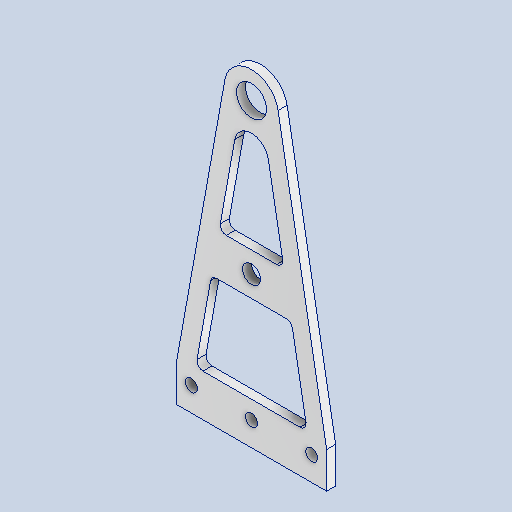
# Autodesk Inventor part: 1171
Saved by Autodesk Inventor 2025.1 (Build 291241000, 241)
## iProperties
Created: 2024-06-11
Part Number: 1171
Material: Aluminium 6061
Document SubType Name: Modeling
Designer: ffogue
Density: 2.7 g/cm^3
Appearance: Aluminium - flach
Author: ffogue
Autodesk Inventor part; units mm, degrees
ref_plane "YZ Plane" through (0, 0, 0) normal (1, 0, 0) x (0, 1, 0)
ref_plane "XZ Plane" through (0, 0, 0) normal (0, 1, 0) x (-1, 0, 0)
ref_plane "XY Plane" through (0, 0, 0) normal (0, 0, 1) x (1, 0, 0)
sketch "Skizze1" plane through (0, 0, 0) normal (0, 1, 0) x (-1, 0, 0)
  line L0 (25, 0) -> (-25, 0)
  line L1 (-25, 0) -> (-25, 12)
  line L2 (-25, 12) -> (-8.8574, 101.5958)
  arc A0 (8.8574, 101.5958) -> (-8.8574, 101.5958) centre (0, 100) ccw
  line L3 (8.8574, 101.5958) -> (25, 12)
  line L4 (25, 12) -> (25, 0)
  line L5 (0, 100) -> (0, 0) construction
  dimension "d0" = 100
  dimension "d1" = 12
  dimension "d2" = 50
  dimension "d3" = 9
  constraints: 12 end point, 2 point on circle, 1 centre point, 1 horizontal, 1 horizontal alignment, 1 midpoint, 1 parallel, 1 perpendicular, 1 symmetric about line, 1 tangent, 1 vertical, 1 vertical alignment
  measures "d0" distance of L5.start L5.end
  measures "d1" distance of L0.end L1.end
  measures "d2" distance of L0.start L0.end
  measures "d3" radius of A0
extrude "Extrusion1" add sketch "Skizze1" along normal blind 3
sketch "Skizze3" plane through (0, 3, 0) normal (0, 1, 0) x (1, 0, 0)
  arc A0 (-8.8574, -101.5958) -> (8.8574, -101.5958) centre (0, -100) ccw projected
  point P0 (0, 0)
  point P1 (0, -100)
  constraints: 1 coincident
hole "Bohrung1" at (0, 3, 100) direction (0, -1, 0) diameter 10 depth 3
sketch "Skizze4" plane through (0, 3, 0) normal (0, 1, 0) x (1, 0, 0)
  line L0 (-10.7957, -57) -> (10.7957, -57)
  line L1 (10.7957, -57) -> (5.5701, -86.0036)
  arc A0 (-5.5701, -86.0036) -> (5.5701, -86.0036) centre (0, -85) ccw
  line L2 (-5.5701, -86.0036) -> (-10.7957, -57)
  line L3 (25, 0) -> (-25, 0) projected
  line L4 (8.8574, -101.5958) -> (25, -12) projected
  line L5 (-25, -12) -> (-8.8574, -101.5958) projected
  circle A1 centre (0, -100) radius 5 projected
  point P0 (0, 0)
  point P1 (0, 0)
  dimension "d13" = 15
  dimension "d14" = 6
  dimension "d15" = 43
  constraints: 6 end point, 2 parallel, 2 point on circle, 1 centre point, 1 horizontal, 1 horizontal alignment, 1 midpoint, 1 tangent, 1 vertical alignment
  measures "d13" distance of A1.centre A0.centre
  measures "d14" distance between parallel lines of L5 L2
  measures "d15" distance from line of L0 A1.centre
extrude "Extrusion2" cut sketch "Skizze4" against normal up to surface (3 mm away) contours L0 L1 A0 L2
sketch "Skizze5" plane through (0, 3, 0) normal (0, 1, 0) x (1, 0, 0)
  line L0 (13.3181, -43) -> (-13.3181, -43)
  line L1 (-13.3181, -43) -> (-18.543, -14)
  line L2 (-18.543, -14) -> (18.543, -14)
  line L3 (18.543, -14) -> (13.3181, -43)
  line L4 (8.8574, -101.5958) -> (25, -12) projected
  line L5 (-25, -12) -> (-8.8574, -101.5958) projected
  line L6 (25, 0) -> (-25, 0) projected
  line L7 (-10.7957, -57) -> (10.7957, -57) projected
  point P0 (0, 0)
  point P1 (0, -14)
  point P2 (0, 0)
  dimension "d18" = 6
  dimension "d19" = 14
  dimension "d20" = 14
  constraints: 8 end point, 3 parallel, 2 midpoint, 1 horizontal, 1 vertical alignment
  measures "d18" distance between parallel lines of L4 L3
  measures "d19" distance between parallel lines of L0 L7
  measures "d20" distance between parallel lines of L6 L2
extrude "Extrusion3" cut sketch "Skizze5" against normal up to surface (3 mm away)
sketch "Skizze6" plane through (0, 3, 0) normal (0, 1, 0) x (1, 0, 0)
  line L0 (25, 0) -> (-25, 0) projected
  line L1 (-10.7957, -57) -> (10.7957, -57) projected
  point P0 (0, 0)
  point P1 (0, -50)
  point P2 (0, 0)
  dimension "d30" = 7
  constraints: 1 midpoint, 1 vertical alignment
  measures "d30" distance from line of point (0, -50) L1
hole "Bohrung2" at (0, 3, 50) direction (0, -1, 0) diameter 6 end through all
fillet "Rundung1" radius 2 6 edges at (10.7957, 1.5, 57) (-10.7957, 1.5, 57) (-13.3181, 1.5, 43) (13.3181, 1.5, 43) (18.543, 1.5, 14) (-18.543, 1.5, 14)
sketch "Skizze7" plane through (0, 3, 0) normal (0, 1, 0) x (1, 0, 0)
  line L0 (25, -12) -> (25, 0) projected
  line L1 (-25, 0) -> (-25, -12) projected
  line L2 (25, 0) -> (-25, 0) projected
  point P0 (0, 0)
  point P1 (20, -8)
  point P2 (0, -8)
  point P3 (-20, -8)
  dimension "d39" = 5
  dimension "d40" = 5
  dimension "d41" = 20
  dimension "d42" = 8
  constraints: 2 horizontal alignment
  measures "d39" distance from line of L0 point (20, -8)
  measures "d40" distance from line of L1 point (-20, -8)
  measures "d41" distance of point (0, -8) point (20, -8)
  measures "d42" distance from line of L2 point (20, -8)
hole "Bohrung3" at (20, 3, 8) at (0, 3, 8) at (-20, 3, 8) direction (0, -1, 0) diameter 4 end through all
